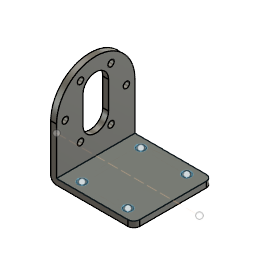
jgb37_motor_bracket_v0_1 (Autodesk Fusion 360 design; units mm, degrees)
part number: 2026-05-27-16-46-23-525
Autodesk Fusion 360 part; units mm, degrees
sketch "草图1" plane through (0, 0, 0) normal (0, 1, 0) x (1, 0, 0)
  line L0 (0, 0) -> (36.4, 0)
  line L1 (39.4, 3) -> (39.4, 37)
  line L2 (36.4, 40) -> (0, 40)
  line L3 (0, 40) -> (0, 0)
  arc A0 (36.4, 0) -> (39.4, 3) centre (36.4, 3) ccw
  arc A1 (39.4, 37) -> (36.4, 40) centre (36.4, 37) ccw
  point P0 (39.4, 0)
  point P1 (39.4, 40)
  dimension "d1" = 39.4
  dimension "d2" = 40
  dimension "d3" = 3
  dimension "d4" = 3
  constraint horizontal L0
  constraint vertical L1
  constraint horizontal L2
  constraint vertical L3
  constraint coincident L0.start L3.end
  constraint coincident P0 L0
  constraint coincident P0 L1
  constraint tangent L0 A0
  constraint tangent L1 A0
  constraint coincident P1 L1
  constraint coincident P1 L2
  constraint tangent L1 A1
  constraint tangent L2 A1
  measures "d1" distance of L0.start P0
  measures "d2" distance of P0 P1
  measures "d3" radius of A0
  measures "d4" radius of A1
sketch "草图2" plane through (0, 0, 0) normal (1, 0, 0) x (0, 0, -1)
  line L0 (0, 0) -> (40, 0)
  line L1 (40, 0) -> (40, 27)
  line L2 (0, 27) -> (0, 0)
  arc A0 (40, 27) -> (0, 27) centre (20, 27) ccw
  line L3 (20, 60) -> (20, -25) construction
  line L4 (40, 26.5) -> (0, 26.5) construction
  line L5 (20, 40) -> (20, 13)
  line L6 (26.5, 33.5) -> (26.5, 19.5)
  line L7 (13.5, 33.5) -> (13.5, 19.5)
  arc A1 (26.5, 33.5) -> (13.5, 33.5) centre (20, 33.5) ccw
  arc A2 (13.5, 19.5) -> (26.5, 19.5) centre (20, 19.5) ccw
  circle A3 centre (4.4115, 26.5) radius 1.6
  circle A4 centre (12.2058, 13) radius 1.6
  circle A5 centre (27.7942, 13) radius 1.6
  circle A6 centre (35.5885, 26.5) radius 1.6
  circle A7 centre (27.7942, 40) radius 1.6
  circle A8 centre (12.2058, 40) radius 1.6
  line L8 (40, 0) -> (0, 0)
  point P0 (0, 26.5)
  point P1 (40, 26.5)
  point P2 (20, 26.5)
  dimension "d5" = 40
  dimension "d6" = 27
  dimension "d7" = 0.5
  dimension "d8" = 27
  dimension "d11" = 13
  dimension "d12" = 3.2
  dimension "d14" = 360
  dimension "d15" = 13
  constraint horizontal L0
  constraint vertical L1
  constraint vertical L2
  constraint coincident L0.start L2.end
  constraint tangent L2 A0
  constraint perpendicular L0 L3
  constraint equal L1 L2
  constraint coincident L2 P0
  constraint coincident L1 P1
  constraint symmetric L3 P0 P1
  constraint coincident P1 L4.start
  constraint coincident P0 L4.end
  constraint coincident L3 L5.start
  constraint perpendicular L4 L5
  constraint symmetric L4 L5.start L5.end
  constraint coincident L5 A1.centre
  constraint symmetric L4 L6.start L6.end
  constraint symmetric L4 L7.start L7.end
  constraint symmetric L4 A1 A2
  constraint midpoint L5 P2
  constraint coincident L4 A3.centre
  measures "d5" distance of L0.start L0.end
  measures "d6" distance of L0.start L2.start
  measures "d7" distance of L2.start P0
  measures "d8" distance of L5.start L5.end
  measures "d11" distance of L6.start L7.start
  measures "d12" diameter of A3
  measures "d15" distance of A4.centre L8
extrude "拉伸1" add sketch "草图1" along normal blind 3
extrude "拉伸2" add sketch "草图2" against normal blind 3
sketch "草图4" plane through (0, 3, 0) normal (0, 1, 0) x (-1, 0, 0)
  arc A0 (-39.4, -37) -> (-36.4, -40) centre (-36.4, -37) ccw
  line L0 (-36.4, -40) -> (0, -40)
  line L1 (0, -40) -> (0, 0)
  line L2 (0, 0) -> (-36.4, 0)
  arc A1 (-36.4, 0) -> (-39.4, -3) centre (-36.4, -3) ccw
  line L3 (-39.4, -3) -> (-39.4, -37)
  circle A2 centre (-31.4, -5) radius 2
  line L4 (20, -20) -> (-52.8436, -20) construction
  circle A3 centre (-31.4, -35) radius 2
  circle A4 centre (-8, -5) radius 2
  circle A5 centre (-8, -35) radius 2
  dimension "d36" = 4
  dimension "d37" = 8
  dimension "d38" = 30
  dimension "d39" = 23.4
  constraint horizontal L4
  constraint equal A2 A3
  constraint symmetric A2.centre L4 A3.centre
  constraint equal A2 A4
  constraint equal A2 A5
  constraint symmetric L4 A4 A5
  measures "d36" diameter of A2
  measures "d37" distance of L3 A2.centre
  measures "d38" distance of A2.centre A3.centre
  measures "d39" distance of A2.centre A4.centre
extrude "拉伸7" cut sketch "草图4" against normal blind 3 contours A4
extrude "拉伸8" cut sketch "草图4" against normal blind 3 contours A2
extrude "拉伸9" cut sketch "草图4" against normal blind 3 contours A3 | A5
fillet "圆角2" radius 3 1 edges at (-3, 0, -20)
sketch "草图3" plane through (0, 3, 0) normal (0, 1, 0) x (-1, 0, 0)
  arc A0 (-39.4, -37) -> (-36.4, -40) centre (-36.4, -37) ccw
  line L0 (-36.4, -40) -> (0, -40)
  line L1 (0, -40) -> (0, 0)
  line L2 (0, 0) -> (-36.4, 0)
  arc A1 (-36.4, 0) -> (-39.4, -3) centre (-36.4, -3) ccw
  line L3 (-39.4, -3) -> (-39.4, -37)
  circle A2 centre (-29.9, -5) radius 2
  circle A3 centre (-6.5, -35) radius 2
  circle A4 centre (-29.9, -35) radius 2
  circle A5 centre (-6.5, -5) radius 2
  line L4 (-18.2, -40) -> (-18.2, 0) construction
  line L5 (-39.4, -20) -> (0, -20) construction
  point P0 (-18.2, -40)
  point P1 (-39.4, -20)
  dimension "d20" = 4
  dimension "d24" = 23.4
  dimension "d25" = 30
  constraint coincident L0 P0
  constraint coincident L3 P1
  constraint midpoint L0 P0
  constraint midpoint L3 P1
  constraint coincident P0 L4.start
  constraint midpoint L2 L4.end
  constraint coincident P1 L5.start
  constraint midpoint L1 L5.end
  constraint symmetric A2.centre A5.centre L4
  constraint equal A2 A3
  constraint equal A4 A5
  constraint symmetric A2.centre A4.centre L5
  constraint equal A2 A5
  constraint symmetric A3 A5 L5
  constraint symmetric A3 A4 L4
  measures "d20" diameter of A2
  measures "d24" distance of A2.centre A5.centre
  measures "d25" distance of A2.centre A4.centre
extrude "拉伸3" [rolled back] along distance -3 taper angle 0
extrude "拉伸4" [rolled back] along distance -3 taper angle 0
extrude "拉伸5" [rolled back] along distance -3 taper angle 0
extrude "拉伸6" [rolled back] along distance -3 taper angle 0
fillet "圆角1" [rolled back] radius 3
